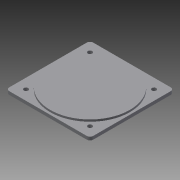
# Autodesk Inventor part: 3-125-instrument-blank
Saved by Autodesk Inventor 2015 (Build 190159000, 159)
## iProperties
Created: 2016-01-17
Part Number: 3-125-instrument-blank
Material: Generic
Document SubType Name: Modeling
Designer: bovine
Density: 1 g/cm^3
Appearance: Default
Author: bovine
Autodesk Inventor part; units mm, degrees
ref_plane "YZ Plane" through (0, 0, 0) normal (1, 0, 0) x (0, 1, 0)
ref_plane "XZ Plane" through (0, 0, 0) normal (0, 1, 0) x (-1, 0, 0)
ref_plane "XY Plane" through (0, 0, 0) normal (0, 0, 1) x (1, 0, 0)
sketch "Sketch1" plane through (0, 0, 0) normal (0, 1, 0) x (-1, 0, 0)
  line L0 (41.275, 41.275) -> (-41.275, 41.275)
  line L1 (-41.275, 41.275) -> (-41.275, -41.275)
  line L2 (-41.275, -41.275) -> (41.275, -41.275)
  line L3 (41.275, -41.275) -> (41.275, 41.275)
  circle A0 centre (0, 0) radius 44.45 construction
  circle A1 centre (0, 0) radius 39.6875
  line L4 (-41.275, 41.275) -> (41.275, -41.275) construction
  line L5 (41.275, 41.275) -> (-41.275, -41.275) construction
  circle A2 centre (31.4309, 31.4309) radius 2.159
  circle A3 centre (31.4309, -31.4309) radius 2.159
  circle A4 centre (-31.4309, 31.4309) radius 2.159
  circle A5 centre (-31.4309, -31.4309) radius 2.159
  point P0 (0, 0)
  point P1 (0, 0)
  point P2 (0, 0)
  dimension "d0" = 82.55
  dimension "d1" = 82.55
  dimension "d2" = 88.9
  dimension "d3" = 79.375
  dimension "d4" = 4.318
  dimension "d5" = 4.318
  dimension "d6" = 4.318
  dimension "d7" = 4.318
  constraints: 12 end point, 6 centre point, 4 coincident, 4 point on circle, 4 point on line, 2 midpoint, 2 parallel, 1 horizontal, 1 perpendicular
  measures "d0" distance of L2.end L1.end
  measures "d1" distance of L1.end L0.end
  measures "d2" diameter of A0
  measures "d3" diameter of A1
  measures "d4" diameter of A2
  measures "d5" diameter of A3
  measures "d6" diameter of A4
  measures "d7" diameter of A5
extrude "Extrusion1" add sketch "Sketch1" along normal blind 3.175 contours L3 L2 L1 L0 | A1
sketch "Sketch2" plane through (0, 3.175, 0) normal (0, 1, 0) x (1, 0, 0)
  circle A0 centre (0, 0) radius 39.0525
  circle A1 centre (0, 0) radius 39.6875 construction
  point P0 (0, 0)
  dimension "d10" = 78.105
  dimension "d17" = 79.375
  constraints: 2 centre point, 2 coincident
  measures "d10" diameter of A0
  measures "d17" diameter of A1
extrude "Extrusion2" add sketch "Sketch2" along normal blind 1.905
fillet "Fillet1" radius 3.175 1 edges at (41.275, 1.5875, 41.275)
fillet "Fillet2" radius 3.175 1 edges at (-41.275, 1.5875, 41.275)
fillet "Fillet3" radius 3.175 1 edges at (41.275, 1.5875, -41.275)
fillet "Fillet4" radius 3.175 1 edges at (-41.275, 1.5875, -41.275)
body "Solid1"
